Autodesk Inventor part; units mm, degrees
(part 6 of 7)
sketch "スケッチ11" plane through (148.5, 105, 2.25) normal (0, 0, 1) x (1, 0, 0)
  circle A0 centre (0, 0) radius 2 projected
  circle A1 centre (0, 0) radius 6 projected
  circle A2 centre (0, 0) radius 18.25 projected
  arc A3 (0.4109, 20.0429) -> (0.2771, 19.6719) centre (6.369, 17.6849) ccw projected
  arc A4 (0.6052, 20.4911) -> (0.4109, 20.0429) centre (7.4658, 17.2508) ccw projected
  arc A5 (1.0044, 20.4754) -> (0.6052, 20.4911) centre (0, 0) ccw projected
  arc A6 (1.1629, 20.0133) -> (1.0044, 20.4754) centre (-6.0894, 17.7834) ccw projected
  arc A7 (1.2671, 19.633) -> (1.1629, 20.0133) centre (-4.9618, 18.1301) ccw projected
  arc A8 (1.331, 19.3292) -> (1.2671, 19.633) centre (-3.8577, 18.3965) ccw projected
  arc A9 (1.7091, 19.2995) -> (1.331, 19.3292) centre (0, 0) ccw projected
  arc A10 (1.8197, 19.5895) -> (1.7091, 19.2995) centre (6.6881, 17.5665) ccw projected
  arc A11 (1.9822, 19.9489) -> (1.8197, 19.5895) centre (7.7369, 17.1307) ccw projected
  arc A12 (2.2111, 20.3804) -> (1.9822, 19.9489) centre (8.7963, 16.6119) ccw projected
  arc A13 (2.6078, 20.3335) -> (2.2111, 20.3804) centre (0, 0) ccw projected
  arc A14 (2.7295, 19.8604) -> (2.6078, 20.3335) centre (-4.6753, 18.2064) ccw projected
  arc A15 (2.8036, 19.473) -> (2.7295, 19.8604) centre (-3.5241, 18.4635) ccw projected
  arc A16 (2.8435, 19.1652) -> (2.8036, 19.473) centre (-2.4025, 18.6425) ccw projected
  arc A17 (3.2181, 19.1059) -> (2.8435, 19.1652) centre (0, 0) ccw projected
  arc A18 (3.3511, 19.3863) -> (3.2181, 19.1059) centre (8.0457, 16.9876) ccw projected
  arc A19 (3.5413, 19.7318) -> (3.3511, 19.3863) centre (9.0571, 16.4708) ccw projected
  arc A20 (3.8033, 20.1441) -> (3.5413, 19.7318) centre (10.0726, 15.8705) ccw projected
  arc A21 (4.1951, 20.0662) -> (3.8033, 20.1441) centre (0, 0) ccw projected
  arc A22 (4.2793, 19.585) -> (4.1951, 20.0662) centre (-3.2324, 18.517) ccw projected
  arc A23 (4.3228, 19.193) -> (4.2793, 19.585) centre (-2.0646, 18.6831) ccw projected
  arc A24 (4.3384, 18.883) -> (4.3228, 19.193) centre (-0.9324, 18.7735) ccw projected
  arc A25 (4.7072, 18.7945) -> (4.3384, 18.883) centre (0, 0) ccw projected
  arc A26 (4.8618, 19.0636) -> (4.7072, 18.7945) centre (9.3537, 16.304) ccw projected
  arc A27 (5.0785, 19.3932) -> (4.8618, 19.0636) centre (10.3215, 15.7095) ccw projected
  arc A28 (5.372, 19.7836) -> (5.0785, 19.3932) centre (11.2867, 15.0313) ccw projected
  arc A29 (5.7565, 19.6752) -> (5.372, 19.7836) centre (0, 0) ccw projected
  arc A30 (5.8028, 19.1889) -> (5.7565, 19.6752) centre (-1.7696, 18.7136) ccw projected
  arc A31 (5.8154, 18.7947) -> (5.8028, 19.1889) centre (-0.5924, 18.7875) ccw projected
  arc A32 (5.8066, 18.4844) -> (5.8154, 18.7947) centre (0.5434, 18.7888) ccw projected
  arc A33 (6.1673, 18.3672) -> (5.8066, 18.4844) centre (0, 0) ccw projected
  arc A34 (6.3425, 18.6234) -> (6.1673, 18.3672) centre (10.6041, 15.5199) ccw projected
  arc A35 (6.5844, 18.9349) -> (6.3425, 18.6234) centre (11.5222, 14.8512) ccw projected
  arc A36 (6.9077, 19.3011) -> (6.5844, 18.9349) centre (12.4312, 14.0994) ccw projected
  arc A37 (7.2825, 19.1629) -> (6.9077, 19.3011) centre (0, 0) ccw projected
  arc A38 (7.2904, 18.6745) -> (7.2825, 19.1629) centre (-0.2959, 18.7947) ccw projected
  arc A39 (7.272, 18.2805) -> (7.2904, 18.6745) centre (0.8835, 18.776) ccw projected
  arc A40 (7.2389, 17.9719) -> (7.272, 18.2805) centre (2.0159, 18.6882) ccw projected
  arc A41 (7.5893, 17.8267) -> (7.2389, 17.9719) centre (0, 0) ccw projected
  arc A42 (7.7842, 18.0684) -> (7.5893, 17.8267) centre (11.7891, 14.64) ccw projected
  arc A43 (8.0497, 18.36) -> (7.7842, 18.0684) centre (12.6519, 13.9014) ccw projected
  arc A44 (8.4007, 18.6997) -> (8.0497, 18.36) centre (13.4991, 13.0806) ccw projected
  arc A45 (8.7635, 18.5324) -> (8.4007, 18.6997) centre (0, 0) ccw projected
  arc A46 (8.7331, 18.0449) -> (8.7635, 18.5324) centre (1.1796, 18.76) ccw projected
  arc A47 (8.6839, 17.6536) -> (8.7331, 18.0449) centre (2.3539, 18.6488) ccw projected
  arc A48 (8.6267, 17.3485) -> (8.6839, 17.6536) centre (3.476, 18.4724) ccw projected
  arc A49 (8.9646, 17.1763) -> (8.6267, 17.3485) centre (0, 0) ccw projected
  arc A50 (9.1778, 17.4019) -> (8.9646, 17.1763) centre (12.9014, 13.6699) ccw projected
  arc A51 (9.4654, 17.6718) -> (9.1778, 17.4019) centre (13.7036, 12.8659) ccw projected
  arc A52 (9.842, 17.9829) -> (9.4654, 17.6718) centre (14.4838, 11.9812) ccw projected
  arc A53 (10.1905, 17.7877) -> (9.842, 17.9829) centre (0, 0) ccw projected
  arc A54 (10.122, 17.3041) -> (10.1905, 17.7877) centre (2.6478, 18.6096) ccw projected
  arc A55 (10.0422, 16.9178) -> (10.122, 17.3041) centre (3.8099, 18.4067) ccw projected
  arc A56 (9.9612, 16.6182) -> (10.0422, 16.9178) centre (4.9146, 18.1428) ccw projected
  arc A57 (10.2846, 16.42) -> (9.9612, 16.6182) centre (0, 0) ccw projected
  arc A58 (10.5148, 16.6282) -> (10.2846, 16.42) centre (13.9341, 12.6156) ccw projected
  arc A59 (10.8227, 16.8747) -> (10.5148, 16.6282) centre (14.6708, 11.7511) ccw projected
  arc A60 (11.2226, 17.1553) -> (10.8227, 16.8747) centre (15.3792, 10.8078) ccw projected
  arc A61 (11.5547, 16.9334) -> (11.2226, 17.1553) centre (0, 0) ccw projected
  arc A62 (11.4485, 16.4566) -> (11.5547, 16.9334) centre (4.0998, 18.3445) ccw projected
  arc A63 (11.3386, 16.0778) -> (11.4485, 16.4566) centre (5.2423, 18.051) ccw projected
  arc A64 (11.2344, 15.7854) -> (11.3386, 16.0778) centre (6.3229, 17.7012) ccw projected
  arc A65 (11.5412, 15.5625) -> (11.2344, 15.7854) centre (0, 0) ccw projected
  arc A66 (11.7871, 15.752) -> (11.5412, 15.5625) centre (14.881, 11.4834) ccw projected
  arc A67 (12.1134, 15.9735) -> (11.7871, 15.752) centre (15.5476, 10.5638) ccw projected
  arc A68 (12.534, 16.2219) -> (12.1134, 15.9735) centre (16.1798, 9.5679) ccw projected
  arc A69 (12.8477, 15.9746) -> (12.534, 16.2219) centre (0, 0) ccw projected
  arc A70 (12.7043, 15.5076) -> (12.8477, 15.9746) centre (5.5264, 17.9663) ccw projected
  arc A71 (12.5651, 15.1386) -> (12.7043, 15.5076) centre (6.6424, 17.5841) ccw projected
  arc A72 (12.4383, 14.8553) -> (12.5651, 15.1386) centre (7.6922, 17.1506) ccw projected
  arc A73 (12.7266, 14.609) -> (12.4383, 14.8553) centre (0, 0) ccw projected
  arc A74 (12.9866, 14.7786) -> (12.7266, 14.609) centre (15.7361, 10.2805) ccw projected
  arc A75 (13.3293, 14.9739) -> (12.9866, 14.7786) centre (16.3285, 9.3114) ccw projected
  arc A76 (13.7681, 15.1885) -> (13.3293, 14.9739) centre (16.8806, 8.2689) ccw projected
  arc A77 (14.0614, 14.9173) -> (13.7681, 15.1885) centre (0, 0) ccw projected
  arc A78 (13.8819, 14.463) -> (14.0614, 14.9173) centre (6.919, 17.4773) ccw projected
  arc A79 (13.7141, 14.1061) -> (13.8819, 14.463) centre (8.0015, 17.0087) ccw projected
  arc A80 (13.5655, 13.8336) -> (13.7141, 14.1061) centre (9.0141, 16.4942) ccw projected
  arc A81 (13.8336, 13.5655) -> (13.5655, 13.8336) centre (0, 0) ccw projected
  arc A82 (14.1061, 13.7141) -> (13.8336, 13.5655) centre (16.4942, 9.0141) ccw projected
  arc A83 (14.463, 13.8819) -> (14.1061, 13.7141) centre (17.0087, 8.0015) ccw projected
  arc A84 (14.9173, 14.0614) -> (14.463, 13.8819) centre (17.4773, 6.919) ccw projected
  arc A85 (15.1885, 13.7681) -> (14.9173, 14.0614) centre (0, 0) ccw projected
  arc A86 (14.9739, 13.3293) -> (15.1885, 13.7681) centre (8.2689, 16.8806) ccw projected
  arc A87 (14.7786, 12.9866) -> (14.9739, 13.3293) centre (9.3114, 16.3285) ccw projected
  arc A88 (14.609, 12.7266) -> (14.7786, 12.9866) centre (10.2805, 15.7361) ccw projected
  arc A89 (14.8553, 12.4383) -> (14.609, 12.7266) centre (0, 0) ccw projected
  arc A90 (15.1386, 12.5651) -> (14.8553, 12.4383) centre (17.1506, 7.6922) ccw projected
  arc A91 (15.5076, 12.7043) -> (15.1386, 12.5651) centre (17.5841, 6.6424) ccw projected
  arc A92 (15.9746, 12.8477) -> (15.5076, 12.7043) centre (17.9663, 5.5264) ccw projected
  arc A93 (16.2219, 12.534) -> (15.9746, 12.8477) centre (0, 0) ccw projected
  arc A94 (15.9735, 12.1134) -> (16.2219, 12.534) centre (9.5679, 16.1798) ccw projected
  arc A95 (15.752, 11.7871) -> (15.9735, 12.1134) centre (10.5638, 15.5476) ccw projected
  arc A96 (15.5625, 11.5412) -> (15.752, 11.7871) centre (11.4834, 14.881) ccw projected
  arc A97 (15.7854, 11.2344) -> (15.5625, 11.5412) centre (0, 0) ccw projected
  arc A98 (16.0778, 11.3386) -> (15.7854, 11.2344) centre (17.7012, 6.3229) ccw projected
  arc A99 (16.4566, 11.4485) -> (16.0778, 11.3386) centre (18.051, 5.2423) ccw projected
  arc A100 (16.9334, 11.5547) -> (16.4566, 11.4485) centre (18.3445, 4.0998) ccw projected
  arc A101 (17.1553, 11.2226) -> (16.9334, 11.5547) centre (0, 0) ccw projected
  arc A102 (16.8747, 10.8227) -> (17.1553, 11.2226) centre (10.8078, 15.3792) ccw projected
  arc A103 (16.6282, 10.5148) -> (16.8747, 10.8227) centre (11.7511, 14.6708) ccw projected
  arc A104 (16.42, 10.2846) -> (16.6282, 10.5148) centre (12.6156, 13.9341) ccw projected
  arc A105 (16.6182, 9.9612) -> (16.42, 10.2846) centre (0, 0) ccw projected
  arc A106 (16.9178, 10.0422) -> (16.6182, 9.9612) centre (18.1428, 4.9146) ccw projected
  arc A107 (17.3041, 10.122) -> (16.9178, 10.0422) centre (18.4067, 3.8099) ccw projected
  arc A108 (17.7877, 10.1905) -> (17.3041, 10.122) centre (18.6096, 2.6478) ccw projected
  arc A109 (17.9829, 9.842) -> (17.7877, 10.1905) centre (0, 0) ccw projected
  arc A110 (17.6718, 9.4654) -> (17.9829, 9.842) centre (11.9812, 14.4838) ccw projected
  arc A111 (17.4019, 9.1778) -> (17.6718, 9.4654) centre (12.8659, 13.7036) ccw projected
  arc A112 (17.1763, 8.9646) -> (17.4019, 9.1778) centre (13.6699, 12.9014) ccw projected
  arc A113 (17.3485, 8.6267) -> (17.1763, 8.9646) centre (0, 0) ccw projected
  arc A114 (17.6536, 8.6839) -> (17.3485, 8.6267) centre (18.4724, 3.476) ccw projected
  arc A115 (18.0449, 8.7331) -> (17.6536, 8.6839) centre (18.6488, 2.3539) ccw projected
  arc A116 (18.5324, 8.7635) -> (18.0449, 8.7331) centre (18.76, 1.1796) ccw projected
  arc A117 (18.6997, 8.4007) -> (18.5324, 8.7635) centre (0, 0) ccw projected
  arc A118 (18.36, 8.0497) -> (18.6997, 8.4007) centre (13.0806, 13.4991) ccw projected
  arc A119 (18.0684, 7.7842) -> (18.36, 8.0497) centre (13.9014, 12.6519) ccw projected
  arc A120 (17.8267, 7.5893) -> (18.0684, 7.7842) centre (14.64, 11.7891) ccw projected
  arc A121 (17.9719, 7.2389) -> (17.8267, 7.5893) centre (0, 0) ccw projected
  arc A122 (18.2805, 7.272) -> (17.9719, 7.2389) centre (18.6882, 2.0159) ccw projected
  arc A123 (18.6745, 7.2904) -> (18.2805, 7.272) centre (18.776, 0.8835) ccw projected
  arc A124 (19.1629, 7.2825) -> (18.6745, 7.2904) centre (18.7947, -0.2959) ccw projected
  arc A125 (19.3011, 6.9077) -> (19.1629, 7.2825) centre (0, 0) ccw projected
  arc A126 (18.9349, 6.5844) -> (19.3011, 6.9077) centre (14.0994, 12.4312) ccw projected
  arc A127 (18.6234, 6.3425) -> (18.9349, 6.5844) centre (14.8512, 11.5222) ccw projected
  arc A128 (18.3672, 6.1673) -> (18.6234, 6.3425) centre (15.5199, 10.6041) ccw projected
  arc A129 (18.4844, 5.8066) -> (18.3672, 6.1673) centre (0, 0) ccw projected
  arc A130 (18.7947, 5.8154) -> (18.4844, 5.8066) centre (18.7888, 0.5434) ccw projected
  arc A131 (19.1889, 5.8028) -> (18.7947, 5.8154) centre (18.7875, -0.5924) ccw projected
  arc A132 (19.6752, 5.7565) -> (19.1889, 5.8028) centre (18.7136, -1.7696) ccw projected
  arc A133 (19.7836, 5.372) -> (19.6752, 5.7565) centre (0, 0) ccw projected
  arc A134 (19.3932, 5.0785) -> (19.7836, 5.372) centre (15.0313, 11.2867) ccw projected
  arc A135 (19.0636, 4.8618) -> (19.3932, 5.0785) centre (15.7095, 10.3215) ccw projected
  arc A136 (18.7945, 4.7072) -> (19.0636, 4.8618) centre (16.304, 9.3537) ccw projected
  arc A137 (18.883, 4.3384) -> (18.7945, 4.7072) centre (0, 0) ccw projected
  arc A138 (19.193, 4.3228) -> (18.883, 4.3384) centre (18.7735, -0.9324) ccw projected
  arc A139 (19.585, 4.2793) -> (19.193, 4.3228) centre (18.6831, -2.0646) ccw projected
  arc A140 (20.0662, 4.1951) -> (19.585, 4.2793) centre (18.517, -3.2324) ccw projected
  arc A141 (20.1441, 3.8033) -> (20.0662, 4.1951) centre (0, 0) ccw projected
  arc A142 (19.7318, 3.5413) -> (20.1441, 3.8033) centre (15.8705, 10.0726) ccw projected
  arc A143 (19.3863, 3.3511) -> (19.7318, 3.5413) centre (16.4708, 9.0571) ccw projected
  arc A144 (19.1059, 3.2181) -> (19.3863, 3.3511) centre (16.9876, 8.0457) ccw projected
  arc A145 (19.1652, 2.8435) -> (19.1059, 3.2181) centre (0, 0) ccw projected
  arc A146 (19.473, 2.8036) -> (19.1652, 2.8435) centre (18.6425, -2.4025) ccw projected
  arc A147 (19.8604, 2.7295) -> (19.473, 2.8036) centre (18.4635, -3.5241) ccw projected
  arc A148 (20.3335, 2.6078) -> (19.8604, 2.7295) centre (18.2064, -4.6753) ccw projected
  arc A149 (20.3804, 2.2111) -> (20.3335, 2.6078) centre (0, 0) ccw projected
  arc A150 (19.9489, 1.9822) -> (20.3804, 2.2111) centre (16.6119, 8.7963) ccw projected
  arc A151 (19.5895, 1.8197) -> (19.9489, 1.9822) centre (17.1307, 7.7369) ccw projected
  arc A152 (19.2995, 1.7091) -> (19.5895, 1.8197) centre (17.5665, 6.6881) ccw projected
  arc A153 (19.3292, 1.331) -> (19.2995, 1.7091) centre (0, 0) ccw projected
  arc A154 (19.633, 1.2671) -> (19.3292, 1.331) centre (18.3965, -3.8577) ccw projected
  arc A155 (20.0133, 1.1629) -> (19.633, 1.2671) centre (18.1301, -4.9618) ccw projected
  arc A156 (20.4754, 1.0044) -> (20.0133, 1.1629) centre (17.7834, -6.0894) ccw projected
  arc A157 (20.4911, 0.6052) -> (20.4754, 1.0044) centre (0, 0) ccw projected
  arc A158 (20.0429, 0.4109) -> (20.4911, 0.6052) centre (17.2508, 7.4658) ccw projected
  arc A159 (19.6719, 0.2771) -> (20.0429, 0.4109) centre (17.6849, 6.369) ccw projected
  arc A160 (19.3741, 0.1896) -> (19.6719, 0.2771) centre (18.0371, 5.2892) ccw projected
  arc A161 (19.3741, -0.1896) -> (19.3741, 0.1896) centre (0, 0) ccw projected
  arc A162 (19.6719, -0.2771) -> (19.3741, -0.1896) centre (18.0371, -5.2892) ccw projected
  arc A163 (20.0429, -0.4109) -> (19.6719, -0.2771) centre (17.6849, -6.369) ccw projected
  arc A164 (20.4911, -0.6052) -> (20.0429, -0.4109) centre (17.2508, -7.4658) ccw projected
  arc A165 (20.4754, -1.0044) -> (20.4911, -0.6052) centre (0, 0) ccw projected
  arc A166 (20.0133, -1.1629) -> (20.4754, -1.0044) centre (17.7834, 6.0894) ccw projected
  arc A167 (19.633, -1.2671) -> (20.0133, -1.1629) centre (18.1301, 4.9618) ccw projected
  arc A168 (19.3292, -1.331) -> (19.633, -1.2671) centre (18.3965, 3.8577) ccw projected
  arc A169 (19.2995, -1.7091) -> (19.3292, -1.331) centre (0, 0) ccw projected
  arc A170 (19.5895, -1.8197) -> (19.2995, -1.7091) centre (17.5665, -6.6881) ccw projected
  arc A171 (19.9489, -1.9822) -> (19.5895, -1.8197) centre (17.1307, -7.7369) ccw projected
  arc A172 (20.3804, -2.2111) -> (19.9489, -1.9822) centre (16.6119, -8.7963) ccw projected
  arc A173 (20.3335, -2.6078) -> (20.3804, -2.2111) centre (0, 0) ccw projected
  arc A174 (19.8604, -2.7295) -> (20.3335, -2.6078) centre (18.2064, 4.6753) ccw projected
  arc A175 (19.473, -2.8036) -> (19.8604, -2.7295) centre (18.4635, 3.5241) ccw projected
  arc A176 (19.1652, -2.8435) -> (19.473, -2.8036) centre (18.6425, 2.4025) ccw projected
  arc A177 (19.1059, -3.2181) -> (19.1652, -2.8435) centre (0, 0) ccw projected
  arc A178 (19.3863, -3.3511) -> (19.1059, -3.2181) centre (16.9876, -8.0457) ccw projected
  arc A179 (19.7318, -3.5413) -> (19.3863, -3.3511) centre (16.4708, -9.0571) ccw projected
  arc A180 (20.1441, -3.8033) -> (19.7318, -3.5413) centre (15.8705, -10.0726) ccw projected
  arc A181 (20.0662, -4.1951) -> (20.1441, -3.8033) centre (0, 0) ccw projected
  arc A182 (19.585, -4.2793) -> (20.0662, -4.1951) centre (18.517, 3.2324) ccw projected
  arc A183 (19.193, -4.3228) -> (19.585, -4.2793) centre (18.6831, 2.0646) ccw projected
  arc A184 (18.883, -4.3384) -> (19.193, -4.3228) centre (18.7735, 0.9324) ccw projected
  arc A185 (18.7945, -4.7072) -> (18.883, -4.3384) centre (0, 0) ccw projected
  arc A186 (19.0636, -4.8618) -> (18.7945, -4.7072) centre (16.304, -9.3537) ccw projected
  arc A187 (19.3932, -5.0785) -> (19.0636, -4.8618) centre (15.7095, -10.3215) ccw projected
  arc A188 (19.7836, -5.372) -> (19.3932, -5.0785) centre (15.0313, -11.2867) ccw projected
  arc A189 (19.6752, -5.7565) -> (19.7836, -5.372) centre (0, 0) ccw projected
  arc A190 (19.1889, -5.8028) -> (19.6752, -5.7565) centre (18.7136, 1.7696) ccw projected
  arc A191 (18.7947, -5.8154) -> (19.1889, -5.8028) centre (18.7875, 0.5924) ccw projected
  arc A192 (18.4844, -5.8066) -> (18.7947, -5.8154) centre (18.7888, -0.5434) ccw projected
  arc A193 (18.3672, -6.1673) -> (18.4844, -5.8066) centre (0, 0) ccw projected
  arc A194 (18.6234, -6.3425) -> (18.3672, -6.1673) centre (15.5199, -10.6041) ccw projected
  arc A195 (18.9349, -6.5844) -> (18.6234, -6.3425) centre (14.8512, -11.5222) ccw projected
  arc A196 (19.3011, -6.9077) -> (18.9349, -6.5844) centre (14.0994, -12.4312) ccw projected
  arc A197 (19.1629, -7.2825) -> (19.3011, -6.9077) centre (0, 0) ccw projected
  arc A198 (18.6745, -7.2904) -> (19.1629, -7.2825) centre (18.7947, 0.2959) ccw projected
  arc A199 (18.2805, -7.272) -> (18.6745, -7.2904) centre (18.776, -0.8835) ccw projected
  arc A200 (17.9719, -7.2389) -> (18.2805, -7.272) centre (18.6882, -2.0159) ccw projected
  arc A201 (17.8267, -7.5893) -> (17.9719, -7.2389) centre (0, 0) ccw projected
  arc A202 (18.0684, -7.7842) -> (17.8267, -7.5893) centre (14.64, -11.7891) ccw projected
  arc A203 (18.36, -8.0497) -> (18.0684, -7.7842) centre (13.9014, -12.6519) ccw projected
  arc A204 (18.6997, -8.4007) -> (18.36, -8.0497) centre (13.0806, -13.4991) ccw projected
  arc A205 (18.5324, -8.7635) -> (18.6997, -8.4007) centre (0, 0) ccw projected
  arc A206 (18.0449, -8.7331) -> (18.5324, -8.7635) centre (18.76, -1.1796) ccw projected
  arc A207 (17.6536, -8.6839) -> (18.0449, -8.7331) centre (18.6488, -2.3539) ccw projected
  arc A208 (17.3485, -8.6267) -> (17.6536, -8.6839) centre (18.4724, -3.476) ccw projected
  arc A209 (17.1763, -8.9646) -> (17.3485, -8.6267) centre (0, 0) ccw projected
  arc A210 (17.4019, -9.1778) -> (17.1763, -8.9646) centre (13.6699, -12.9014) ccw projected
  arc A211 (17.6718, -9.4654) -> (17.4019, -9.1778) centre (12.8659, -13.7036) ccw projected
  arc A212 (17.9829, -9.842) -> (17.6718, -9.4654) centre (11.9812, -14.4838) ccw projected
  arc A213 (17.7877, -10.1905) -> (17.9829, -9.842) centre (0, 0) ccw projected
  arc A214 (17.3041, -10.122) -> (17.7877, -10.1905) centre (18.6096, -2.6478) ccw projected
  arc A215 (16.9178, -10.0422) -> (17.3041, -10.122) centre (18.4067, -3.8099) ccw projected
  arc A216 (16.6182, -9.9612) -> (16.9178, -10.0422) centre (18.1428, -4.9146) ccw projected
  arc A217 (16.42, -10.2846) -> (16.6182, -9.9612) centre (0, 0) ccw projected
  arc A218 (16.6282, -10.5148) -> (16.42, -10.2846) centre (12.6156, -13.9341) ccw projected
  arc A219 (16.8747, -10.8227) -> (16.6282, -10.5148) centre (11.7511, -14.6708) ccw projected
  arc A220 (17.1553, -11.2226) -> (16.8747, -10.8227) centre (10.8078, -15.3792) ccw projected
  arc A221 (16.9334, -11.5547) -> (17.1553, -11.2226) centre (0, 0) ccw projected
  arc A222 (16.4566, -11.4485) -> (16.9334, -11.5547) centre (18.3445, -4.0998) ccw projected
  arc A223 (16.0778, -11.3386) -> (16.4566, -11.4485) centre (18.051, -5.2423) ccw projected
  arc A224 (15.7854, -11.2344) -> (16.0778, -11.3386) centre (17.7012, -6.3229) ccw projected
  arc A225 (15.5625, -11.5412) -> (15.7854, -11.2344) centre (0, 0) ccw projected
  arc A226 (15.752, -11.7871) -> (15.5625, -11.5412) centre (11.4834, -14.881) ccw projected
  arc A227 (15.9735, -12.1134) -> (15.752, -11.7871) centre (10.5638, -15.5476) ccw projected
  arc A228 (16.2219, -12.534) -> (15.9735, -12.1134) centre (9.5679, -16.1798) ccw projected
  arc A229 (15.9746, -12.8477) -> (16.2219, -12.534) centre (0, 0) ccw projected
  arc A230 (15.5076, -12.7043) -> (15.9746, -12.8477) centre (17.9663, -5.5264) ccw projected
  arc A231 (15.1386, -12.5651) -> (15.5076, -12.7043) centre (17.5841, -6.6424) ccw projected
  arc A232 (14.8553, -12.4383) -> (15.1386, -12.5651) centre (17.1506, -7.6922) ccw projected
  arc A233 (14.609, -12.7266) -> (14.8553, -12.4383) centre (0, 0) ccw projected
  arc A234 (14.7786, -12.9866) -> (14.609, -12.7266) centre (10.2805, -15.7361) ccw projected
  arc A235 (14.9739, -13.3293) -> (14.7786, -12.9866) centre (9.3114, -16.3285) ccw projected
  arc A236 (15.1885, -13.7681) -> (14.9739, -13.3293) centre (8.2689, -16.8806) ccw projected
  arc A237 (14.9173, -14.0614) -> (15.1885, -13.7681) centre (0, 0) ccw projected
  arc A238 (14.463, -13.8819) -> (14.9173, -14.0614) centre (17.4773, -6.919) ccw projected
  arc A239 (14.1061, -13.7141) -> (14.463, -13.8819) centre (17.0087, -8.0015) ccw projected
  arc A240 (13.8336, -13.5655) -> (14.1061, -13.7141) centre (16.4942, -9.0141) ccw projected
  arc A241 (13.5655, -13.8336) -> (13.8336, -13.5655) centre (0, 0) ccw projected
  arc A242 (13.7141, -14.1061) -> (13.5655, -13.8336) centre (9.0141, -16.4942) ccw projected
  arc A243 (13.8819, -14.463) -> (13.7141, -14.1061) centre (8.0015, -17.0087) ccw projected
  arc A244 (14.0614, -14.9173) -> (13.8819, -14.463) centre (6.919, -17.4773) ccw projected
  arc A245 (13.7681, -15.1885) -> (14.0614, -14.9173) centre (0, 0) ccw projected
  arc A246 (13.3293, -14.9739) -> (13.7681, -15.1885) centre (16.8806, -8.2689) ccw projected
  arc A247 (12.9866, -14.7786) -> (13.3293, -14.9739) centre (16.3285, -9.3114) ccw projected
  arc A248 (12.7266, -14.609) -> (12.9866, -14.7786) centre (15.7361, -10.2805) ccw projected
  arc A249 (12.4383, -14.8553) -> (12.7266, -14.609) centre (0, 0) ccw projected
  arc A250 (12.5651, -15.1386) -> (12.4383, -14.8553) centre (7.6922, -17.1506) ccw projected
  arc A251 (12.7043, -15.5076) -> (12.5651, -15.1386) centre (6.6424, -17.5841) ccw projected
  arc A252 (12.8477, -15.9746) -> (12.7043, -15.5076) centre (5.5264, -17.9663) ccw projected
  arc A253 (12.534, -16.2219) -> (12.8477, -15.9746) centre (0, 0) ccw projected
  arc A254 (12.1134, -15.9735) -> (12.534, -16.2219) centre (16.1798, -9.5679) ccw projected
  arc A255 (11.7871, -15.752) -> (12.1134, -15.9735) centre (15.5476, -10.5638) ccw projected
  arc A256 (11.5412, -15.5625) -> (11.7871, -15.752) centre (14.881, -11.4834) ccw projected
  arc A257 (11.2344, -15.7854) -> (11.5412, -15.5625) centre (0, 0) ccw projected
  arc A258 (11.3386, -16.0778) -> (11.2344, -15.7854) centre (6.3229, -17.7012) ccw projected
  arc A259 (11.4485, -16.4566) -> (11.3386, -16.0778) centre (5.2423, -18.051) ccw projected
  arc A260 (11.5547, -16.9334) -> (11.4485, -16.4566) centre (4.0998, -18.3445) ccw projected
  arc A261 (11.2226, -17.1553) -> (11.5547, -16.9334) centre (0, 0) ccw projected
  arc A262 (10.8227, -16.8747) -> (11.2226, -17.1553) centre (15.3792, -10.8078) ccw projected
  arc A263 (10.5148, -16.6282) -> (10.8227, -16.8747) centre (14.6708, -11.7511) ccw projected
  arc A264 (10.2846, -16.42) -> (10.5148, -16.6282) centre (13.9341, -12.6156) ccw projected
  arc A265 (9.9612, -16.6182) -> (10.2846, -16.42) centre (0, 0) ccw projected
  arc A266 (10.0422, -16.9178) -> (9.9612, -16.6182) centre (4.9146, -18.1428) ccw projected
  arc A267 (10.122, -17.3041) -> (10.0422, -16.9178) centre (3.8099, -18.4067) ccw projected
  arc A268 (10.1905, -17.7877) -> (10.122, -17.3041) centre (2.6478, -18.6096) ccw projected
  arc A269 (9.842, -17.9829) -> (10.1905, -17.7877) centre (0, 0) ccw projected
  arc A270 (9.4654, -17.6718) -> (9.842, -17.9829) centre (14.4838, -11.9812) ccw projected
  arc A271 (9.1778, -17.4019) -> (9.4654, -17.6718) centre (13.7036, -12.8659) ccw projected
  arc A272 (8.9646, -17.1763) -> (9.1778, -17.4019) centre (12.9014, -13.6699) ccw projected
  arc A273 (8.6267, -17.3485) -> (8.9646, -17.1763) centre (0, 0) ccw projected
  arc A274 (8.6839, -17.6536) -> (8.6267, -17.3485) centre (3.476, -18.4724) ccw projected
  arc A275 (8.7331, -18.0449) -> (8.6839, -17.6536) centre (2.3539, -18.6488) ccw projected
  arc A276 (8.7635, -18.5324) -> (8.7331, -18.0449) centre (1.1796, -18.76) ccw projected
  arc A277 (8.4007, -18.6997) -> (8.7635, -18.5324) centre (0, 0) ccw projected
  arc A278 (8.0497, -18.36) -> (8.4007, -18.6997) centre (13.4991, -13.0806) ccw projected
  arc A279 (7.7842, -18.0684) -> (8.0497, -18.36) centre (12.6519, -13.9014) ccw projected
  arc A280 (7.5893, -17.8267) -> (7.7842, -18.0684) centre (11.7891, -14.64) ccw projected
  arc A281 (7.2389, -17.9719) -> (7.5893, -17.8267) centre (0, 0) ccw projected
  arc A282 (7.272, -18.2805) -> (7.2389, -17.9719) centre (2.0159, -18.6882) ccw projected
  arc A283 (7.2904, -18.6745) -> (7.272, -18.2805) centre (0.8835, -18.776) ccw projected
  arc A284 (7.2825, -19.1629) -> (7.2904, -18.6745) centre (-0.2959, -18.7947) ccw projected
  arc A285 (6.9077, -19.3011) -> (7.2825, -19.1629) centre (0, 0) ccw projected
  arc A286 (6.5844, -18.9349) -> (6.9077, -19.3011) centre (12.4312, -14.0994) ccw projected
  arc A287 (6.3425, -18.6234) -> (6.5844, -18.9349) centre (11.5222, -14.8512) ccw projected
  arc A288 (6.1673, -18.3672) -> (6.3425, -18.6234) centre (10.6041, -15.5199) ccw projected
  arc A289 (5.8066, -18.4844) -> (6.1673, -18.3672) centre (0, 0) ccw projected
  arc A290 (5.8154, -18.7947) -> (5.8066, -18.4844) centre (0.5434, -18.7888) ccw projected
  arc A291 (5.8028, -19.1889) -> (5.8154, -18.7947) centre (-0.5924, -18.7875) ccw projected
  arc A292 (5.7565, -19.6752) -> (5.8028, -19.1889) centre (-1.7696, -18.7136) ccw projected
  arc A293 (5.372, -19.7836) -> (5.7565, -19.6752) centre (0, 0) ccw projected
  arc A294 (5.0785, -19.3932) -> (5.372, -19.7836) centre (11.2867, -15.0313) ccw projected
  arc A295 (4.8618, -19.0636) -> (5.0785, -19.3932) centre (10.3215, -15.7095) ccw projected
  arc A296 (4.7072, -18.7945) -> (4.8618, -19.0636) centre (9.3537, -16.304) ccw projected
  arc A297 (4.3384, -18.883) -> (4.7072, -18.7945) centre (0, 0) ccw projected
  arc A298 (4.3228, -19.193) -> (4.3384, -18.883) centre (-0.9324, -18.7735) ccw projected
  arc A299 (4.2793, -19.585) -> (4.3228, -19.193) centre (-2.0646, -18.6831) ccw projected
  arc A300 (4.1951, -20.0662) -> (4.2793, -19.585) centre (-3.2324, -18.517) ccw projected
  arc A301 (3.8033, -20.1441) -> (4.1951, -20.0662) centre (0, 0) ccw projected
  arc A302 (3.5413, -19.7318) -> (3.8033, -20.1441) centre (10.0726, -15.8705) ccw projected
  arc A303 (3.3511, -19.3863) -> (3.5413, -19.7318) centre (9.0571, -16.4708) ccw projected
  arc A304 (3.2181, -19.1059) -> (3.3511, -19.3863) centre (8.0457, -16.9876) ccw projected
  arc A305 (2.8435, -19.1652) -> (3.2181, -19.1059) centre (0, 0) ccw projected
  arc A306 (2.8036, -19.473) -> (2.8435, -19.1652) centre (-2.4025, -18.6425) ccw projected
  arc A307 (2.7295, -19.8604) -> (2.8036, -19.473) centre (-3.5241, -18.4635) ccw projected
  arc A308 (2.6078, -20.3335) -> (2.7295, -19.8604) centre (-4.6753, -18.2064) ccw projected
  arc A309 (2.2111, -20.3804) -> (2.6078, -20.3335) centre (0, 0) ccw projected
  arc A310 (1.9822, -19.9489) -> (2.2111, -20.3804) centre (8.7963, -16.6119) ccw projected
  arc A311 (1.8197, -19.5895) -> (1.9822, -19.9489) centre (7.7369, -17.1307) ccw projected
  arc A312 (1.7091, -19.2995) -> (1.8197, -19.5895) centre (6.6881, -17.5665) ccw projected
  arc A313 (1.331, -19.3292) -> (1.7091, -19.2995) centre (0, 0) ccw projected
  arc A314 (1.2671, -19.633) -> (1.331, -19.3292) centre (-3.8577, -18.3965) ccw projected
  arc A315 (1.1629, -20.0133) -> (1.2671, -19.633) centre (-4.9618, -18.1301) ccw projected
  arc A316 (1.0044, -20.4754) -> (1.1629, -20.0133) centre (-6.0894, -17.7834) ccw projected
  arc A317 (0.6052, -20.4911) -> (1.0044, -20.4754) centre (0, 0) ccw projected
  arc A318 (0.4109, -20.0429) -> (0.6052, -20.4911) centre (7.4658, -17.2508) ccw projected
  arc A319 (0.2771, -19.6719) -> (0.4109, -20.0429) centre (6.369, -17.6849) ccw projected
  arc A320 (0.1896, -19.3741) -> (0.2771, -19.6719) centre (5.2892, -18.0371) ccw projected
  arc A321 (-0.1896, -19.3741) -> (0.1896, -19.3741) centre (0, 0) ccw projected
  arc A322 (-0.2771, -19.6719) -> (-0.1896, -19.3741) centre (-5.2892, -18.0371) ccw projected
  arc A323 (-0.4109, -20.0429) -> (-0.2771, -19.6719) centre (-6.369, -17.6849) ccw projected
  arc A324 (-0.6052, -20.4911) -> (-0.4109, -20.0429) centre (-7.4658, -17.2508) ccw projected
  arc A325 (-1.0044, -20.4754) -> (-0.6052, -20.4911) centre (0, 0) ccw projected
  arc A326 (-1.1629, -20.0133) -> (-1.0044, -20.4754) centre (6.0894, -17.7834) ccw projected
  arc A327 (-1.2671, -19.633) -> (-1.1629, -20.0133) centre (4.9618, -18.1301) ccw projected
  arc A328 (-1.331, -19.3292) -> (-1.2671, -19.633) centre (3.8577, -18.3965) ccw projected
  arc A329 (-1.7091, -19.2995) -> (-1.331, -19.3292) centre (0, 0) ccw projected
  arc A330 (-1.8197, -19.5895) -> (-1.7091, -19.2995) centre (-6.6881, -17.5665) ccw projected
  arc A331 (-1.9822, -19.9489) -> (-1.8197, -19.5895) centre (-7.7369, -17.1307) ccw projected
  arc A332 (-2.2111, -20.3804) -> (-1.9822, -19.9489) centre (-8.7963, -16.6119) ccw projected
  arc A333 (-2.6078, -20.3335) -> (-2.2111, -20.3804) centre (0, 0) ccw projected
  arc A334 (-2.7295, -19.8604) -> (-2.6078, -20.3335) centre (4.6753, -18.2064) ccw projected
  arc A335 (-2.8036, -19.473) -> (-2.7295, -19.8604) centre (3.5241, -18.4635) ccw projected
  arc A336 (-2.8435, -19.1652) -> (-2.8036, -19.473) centre (2.4025, -18.6425) ccw projected
  arc A337 (-3.2181, -19.1059) -> (-2.8435, -19.1652) centre (0, 0) ccw projected
  arc A338 (-3.3511, -19.3863) -> (-3.2181, -19.1059) centre (-8.0457, -16.9876) ccw projected
  arc A339 (-3.5413, -19.7318) -> (-3.3511, -19.3863) centre (-9.0571, -16.4708) ccw projected
  arc A340 (-3.8033, -20.1441) -> (-3.5413, -19.7318) centre (-10.0726, -15.8705) ccw projected
  arc A341 (-4.1951, -20.0662) -> (-3.8033, -20.1441) centre (0, 0) ccw projected
  arc A342 (-4.2793, -19.585) -> (-4.1951, -20.0662) centre (3.2324, -18.517) ccw projected
  arc A343 (-4.3228, -19.193) -> (-4.2793, -19.585) centre (2.0646, -18.6831) ccw projected
  arc A344 (-4.3384, -18.883) -> (-4.3228, -19.193) centre (0.9324, -18.7735) ccw projected
  arc A345 (-4.7072, -18.7945) -> (-4.3384, -18.883) centre (0, 0) ccw projected
  arc A346 (-4.8618, -19.0636) -> (-4.7072, -18.7945) centre (-9.3537, -16.304) ccw projected
  arc A347 (-5.0785, -19.3932) -> (-4.8618, -19.0636) centre (-10.3215, -15.7095) ccw projected
  arc A348 (-5.372, -19.7836) -> (-5.0785, -19.3932) centre (-11.2867, -15.0313) ccw projected
  arc A349 (-5.7565, -19.6752) -> (-5.372, -19.7836) centre (0, 0) ccw projected
  arc A350 (-5.8028, -19.1889) -> (-5.7565, -19.6752) centre (1.7696, -18.7136) ccw projected
  arc A351 (-5.8154, -18.7947) -> (-5.8028, -19.1889) centre (0.5924, -18.7875) ccw projected
  arc A352 (-5.8066, -18.4844) -> (-5.8154, -18.7947) centre (-0.5434, -18.7888) ccw projected
  arc A353 (-6.1673, -18.3672) -> (-5.8066, -18.4844) centre (0, 0) ccw projected
  arc A354 (-6.3425, -18.6234) -> (-6.1673, -18.3672) centre (-10.6041, -15.5199) ccw projected
  arc A355 (-6.5844, -18.9349) -> (-6.3425, -18.6234) centre (-11.5222, -14.8512) ccw projected
  arc A356 (-6.9077, -19.3011) -> (-6.5844, -18.9349) centre (-12.4312, -14.0994) ccw projected
  arc A357 (-7.2825, -19.1629) -> (-6.9077, -19.3011) centre (0, 0) ccw projected
  arc A358 (-7.2904, -18.6745) -> (-7.2825, -19.1629) centre (0.2959, -18.7947) ccw projected
  arc A359 (-7.272, -18.2805) -> (-7.2904, -18.6745) centre (-0.8835, -18.776) ccw projected
  arc A360 (-7.2389, -17.9719) -> (-7.272, -18.2805) centre (-2.0159, -18.6882) ccw projected
  arc A361 (-7.5893, -17.8267) -> (-7.2389, -17.9719) centre (0, 0) ccw projected
  arc A362 (-7.7842, -18.0684) -> (-7.5893, -17.8267) centre (-11.7891, -14.64) ccw projected
  arc A363 (-8.0497, -18.36) -> (-7.7842, -18.0684) centre (-12.6519, -13.9014) ccw projected
  arc A364 (-8.4007, -18.6997) -> (-8.0497, -18.36) centre (-13.4991, -13.0806) ccw projected
  arc A365 (-8.7635, -18.5324) -> (-8.4007, -18.6997) centre (0, 0) ccw projected
  arc A366 (-8.7331, -18.0449) -> (-8.7635, -18.5324) centre (-1.1796, -18.76) ccw projected
  arc A367 (-8.6839, -17.6536) -> (-8.7331, -18.0449) centre (-2.3539, -18.6488) ccw projected
  arc A368 (-8.6267, -17.3485) -> (-8.6839, -17.6536) centre (-3.476, -18.4724) ccw projected
  arc A369 (-8.9646, -17.1763) -> (-8.6267, -17.3485) centre (0, 0) ccw projected
  arc A370 (-9.1778, -17.4019) -> (-8.9646, -17.1763) centre (-12.9014, -13.6699) ccw projected
  arc A371 (-9.4654, -17.6718) -> (-9.1778, -17.4019) centre (-13.7036, -12.8659) ccw projected
  arc A372 (-9.842, -17.9829) -> (-9.4654, -17.6718) centre (-14.4838, -11.9812) ccw projected
  arc A373 (-10.1905, -17.7877) -> (-9.842, -17.9829) centre (0, 0) ccw projected
  arc A374 (-10.122, -17.3041) -> (-10.1905, -17.7877) centre (-2.6478, -18.6096) ccw projected
  arc A375 (-10.0422, -16.9178) -> (-10.122, -17.3041) centre (-3.8099, -18.4067) ccw projected
  arc A376 (-9.9612, -16.6182) -> (-10.0422, -16.9178) centre (-4.9146, -18.1428) ccw projected
  arc A377 (-10.2846, -16.42) -> (-9.9612, -16.6182) centre (0, 0) ccw projected
  arc A378 (-10.5148, -16.6282) -> (-10.2846, -16.42) centre (-13.9341, -12.6156) ccw projected
  arc A379 (-10.8227, -16.8747) -> (-10.5148, -16.6282) centre (-14.6708, -11.7511) ccw projected
  arc A380 (-11.2226, -17.1553) -> (-10.8227, -16.8747) centre (-15.3792, -10.8078) ccw projected
  arc A381 (-11.5547, -16.9334) -> (-11.2226, -17.1553) centre (0, 0) ccw projected
  arc A382 (-11.4485, -16.4566) -> (-11.5547, -16.9334) centre (-4.0998, -18.3445) ccw projected
  arc A383 (-11.3386, -16.0778) -> (-11.4485, -16.4566) centre (-5.2423, -18.051) ccw projected
  arc A384 (-11.2344, -15.7854) -> (-11.3386, -16.0778) centre (-6.3229, -17.7012) ccw projected
  arc A385 (-11.5412, -15.5625) -> (-11.2344, -15.7854) centre (0, 0) ccw projected
  arc A386 (-11.7871, -15.752) -> (-11.5412, -15.5625) centre (-14.881, -11.4834) ccw projected
  arc A387 (-12.1134, -15.9735) -> (-11.7871, -15.752) centre (-15.5476, -10.5638) ccw projected
  arc A388 (-12.534, -16.2219) -> (-12.1134, -15.9735) centre (-16.1798, -9.5679) ccw projected
  arc A389 (-12.8477, -15.9746) -> (-12.534, -16.2219) centre (0, 0) ccw projected
  arc A390 (-12.7043, -15.5076) -> (-12.8477, -15.9746) centre (-5.5264, -17.9663) ccw projected
  arc A391 (-12.5651, -15.1386) -> (-12.7043, -15.5076) centre (-6.6424, -17.5841) ccw projected
  arc A392 (-12.4383, -14.8553) -> (-12.5651, -15.1386) centre (-7.6922, -17.1506) ccw projected
  arc A393 (-12.7266, -14.609) -> (-12.4383, -14.8553) centre (0, 0) ccw projected
  arc A394 (-12.9866, -14.7786) -> (-12.7266, -14.609) centre (-15.7361, -10.2805) ccw projected
  arc A395 (-13.3293, -14.9739) -> (-12.9866, -14.7786) centre (-16.3285, -9.3114) ccw projected
  arc A396 (-13.7681, -15.1885) -> (-13.3293, -14.9739) centre (-16.8806, -8.2689) ccw projected
  arc A397 (-14.0614, -14.9173) -> (-13.7681, -15.1885) centre (0, 0) ccw projected
  arc A398 (-13.8819, -14.463) -> (-14.0614, -14.9173) centre (-6.919, -17.4773) ccw projected
  arc A399 (-13.7141, -14.1061) -> (-13.8819, -14.463) centre (-8.0015, -17.0087) ccw projected
  arc A400 (-13.5655, -13.8336) -> (-13.7141, -14.1061) centre (-9.0141, -16.4942) ccw projected
  arc A401 (-13.8336, -13.5655) -> (-13.5655, -13.8336) centre (0, 0) ccw projected
  arc A402 (-14.1061, -13.7141) -> (-13.8336, -13.5655) centre (-16.4942, -9.0141) ccw projected
  arc A403 (-14.463, -13.8819) -> (-14.1061, -13.7141) centre (-17.0087, -8.0015) ccw projected
  arc A404 (-14.9173, -14.0614) -> (-14.463, -13.8819) centre (-17.4773, -6.919) ccw projected
  arc A405 (-15.1885, -13.7681) -> (-14.9173, -14.0614) centre (0, 0) ccw projected
  arc A406 (-14.9739, -13.3293) -> (-15.1885, -13.7681) centre (-8.2689, -16.8806) ccw projected
  arc A407 (-14.7786, -12.9866) -> (-14.9739, -13.3293) centre (-9.3114, -16.3285) ccw projected
  arc A408 (-14.609, -12.7266) -> (-14.7786, -12.9866) centre (-10.2805, -15.7361) ccw projected
  arc A409 (-14.8553, -12.4383) -> (-14.609, -12.7266) centre (0, 0) ccw projected
  arc A410 (-15.1386, -12.5651) -> (-14.8553, -12.4383) centre (-17.1506, -7.6922) ccw projected
  arc A411 (-15.5076, -12.7043) -> (-15.1386, -12.5651) centre (-17.5841, -6.6424) ccw projected
  arc A412 (-15.9746, -12.8477) -> (-15.5076, -12.7043) centre (-17.9663, -5.5264) ccw projected
  arc A413 (-16.2219, -12.534) -> (-15.9746, -12.8477) centre (0, 0) ccw projected
  arc A414 (-15.9735, -12.1134) -> (-16.2219, -12.534) centre (-9.5679, -16.1798) ccw projected
  arc A415 (-15.752, -11.7871) -> (-15.9735, -12.1134) centre (-10.5638, -15.5476) ccw projected
  arc A416 (-15.5625, -11.5412) -> (-15.752, -11.7871) centre (-11.4834, -14.881) ccw projected
  arc A417 (-15.7854, -11.2344) -> (-15.5625, -11.5412) centre (0, 0) ccw projected
  arc A418 (-16.0778, -11.3386) -> (-15.7854, -11.2344) centre (-17.7012, -6.3229) ccw projected
  arc A419 (-16.4566, -11.4485) -> (-16.0778, -11.3386) centre (-18.051, -5.2423) ccw projected
  arc A420 (-16.9334, -11.5547) -> (-16.4566, -11.4485) centre (-18.3445, -4.0998) ccw projected
  arc A421 (-17.1553, -11.2226) -> (-16.9334, -11.5547) centre (0, 0) ccw projected
  arc A422 (-16.8747, -10.8227) -> (-17.1553, -11.2226) centre (-10.8078, -15.3792) ccw projected
  arc A423 (-16.6282, -10.5148) -> (-16.8747, -10.8227) centre (-11.7511, -14.6708) ccw projected
  arc A424 (-16.42, -10.2846) -> (-16.6282, -10.5148) centre (-12.6156, -13.9341) ccw projected
  arc A425 (-16.6182, -9.9612) -> (-16.42, -10.2846) centre (0, 0) ccw projected
  arc A426 (-16.9178, -10.0422) -> (-16.6182, -9.9612) centre (-18.1428, -4.9146) ccw projected
  arc A427 (-17.3041, -10.122) -> (-16.9178, -10.0422) centre (-18.4067, -3.8099) ccw projected
  arc A428 (-17.7877, -10.1905) -> (-17.3041, -10.122) centre (-18.6096, -2.6478) ccw projected
  arc A429 (-17.9829, -9.842) -> (-17.7877, -10.1905) centre (0, 0) ccw projected
  arc A430 (-17.6718, -9.4654) -> (-17.9829, -9.842) centre (-11.9812, -14.4838) ccw projected
  arc A431 (-17.4019, -9.1778) -> (-17.6718, -9.4654) centre (-12.8659, -13.7036) ccw projected
  arc A432 (-17.1763, -8.9646) -> (-17.4019, -9.1778) centre (-13.6699, -12.9014) ccw projected
  arc A433 (-17.3485, -8.6267) -> (-17.1763, -8.9646) centre (0, 0) ccw projected
  arc A434 (-17.6536, -8.6839) -> (-17.3485, -8.6267) centre (-18.4724, -3.476) ccw projected
  arc A435 (-18.0449, -8.7331) -> (-17.6536, -8.6839) centre (-18.6488, -2.3539) ccw projected
  arc A436 (-18.5324, -8.7635) -> (-18.0449, -8.7331) centre (-18.76, -1.1796) ccw projected
  arc A437 (-18.6997, -8.4007) -> (-18.5324, -8.7635) centre (0, 0) ccw projected
  arc A438 (-18.36, -8.0497) -> (-18.6997, -8.4007) centre (-13.0806, -13.4991) ccw projected
  arc A439 (-18.0684, -7.7842) -> (-18.36, -8.0497) centre (-13.9014, -12.6519) ccw projected
  arc A440 (-17.8267, -7.5893) -> (-18.0684, -7.7842) centre (-14.64, -11.7891) ccw projected
  arc A441 (-17.9719, -7.2389) -> (-17.8267, -7.5893) centre (0, 0) ccw projected
  arc A442 (-18.2805, -7.272) -> (-17.9719, -7.2389) centre (-18.6882, -2.0159) ccw projected
  arc A443 (-18.6745, -7.2904) -> (-18.2805, -7.272) centre (-18.776, -0.8835) ccw projected
  arc A444 (-19.1629, -7.2825) -> (-18.6745, -7.2904) centre (-18.7947, 0.2959) ccw projected
  arc A445 (-19.3011, -6.9077) -> (-19.1629, -7.2825) centre (0, 0) ccw projected
  arc A446 (-18.9349, -6.5844) -> (-19.3011, -6.9077) centre (-14.0994, -12.4312) ccw projected
  arc A447 (-18.6234, -6.3425) -> (-18.9349, -6.5844) centre (-14.8512, -11.5222) ccw projected
  arc A448 (-18.3672, -6.1673) -> (-18.6234, -6.3425) centre (-15.5199, -10.6041) ccw projected
  arc A449 (-18.4844, -5.8066) -> (-18.3672, -6.1673) centre (0, 0) ccw projected
  arc A450 (-18.7947, -5.8154) -> (-18.4844, -5.8066) centre (-18.7888, -0.5434) ccw projected
  arc A451 (-19.1889, -5.8028) -> (-18.7947, -5.8154) centre (-18.7875, 0.5924) ccw projected
  arc A452 (-19.6752, -5.7565) -> (-19.1889, -5.8028) centre (-18.7136, 1.7696) ccw projected
  arc A453 (-19.7836, -5.372) -> (-19.6752, -5.7565) centre (0, 0) ccw projected
  arc A454 (-19.3932, -5.0785) -> (-19.7836, -5.372) centre (-15.0313, -11.2867) ccw projected
  arc A455 (-19.0636, -4.8618) -> (-19.3932, -5.0785) centre (-15.7095, -10.3215) ccw projected
  arc A456 (-18.7945, -4.7072) -> (-19.0636, -4.8618) centre (-16.304, -9.3537) ccw projected
  arc A457 (-18.883, -4.3384) -> (-18.7945, -4.7072) centre (0, 0) ccw projected
  arc A458 (-19.193, -4.3228) -> (-18.883, -4.3384) centre (-18.7735, 0.9324) ccw projected
  arc A459 (-19.585, -4.2793) -> (-19.193, -4.3228) centre (-18.6831, 2.0646) ccw projected
  arc A460 (-20.0662, -4.1951) -> (-19.585, -4.2793) centre (-18.517, 3.2324) ccw projected
  arc A461 (-20.1441, -3.8033) -> (-20.0662, -4.1951) centre (0, 0) ccw projected
  arc A462 (-19.7318, -3.5413) -> (-20.1441, -3.8033) centre (-15.8705, -10.0726) ccw projected
  arc A463 (-19.3863, -3.3511) -> (-19.7318, -3.5413) centre (-16.4708, -9.0571) ccw projected
  arc A464 (-19.1059, -3.2181) -> (-19.3863, -3.3511) centre (-16.9876, -8.0457) ccw projected
  arc A465 (-19.1652, -2.8435) -> (-19.1059, -3.2181) centre (0, 0) ccw projected
  arc A466 (-19.473, -2.8036) -> (-19.1652, -2.8435) centre (-18.6425, 2.4025) ccw projected
  arc A467 (-19.8604, -2.7295) -> (-19.473, -2.8036) centre (-18.4635, 3.5241) ccw projected
  arc A468 (-20.3335, -2.6078) -> (-19.8604, -2.7295) centre (-18.2064, 4.6753) ccw projected
  arc A469 (-20.3804, -2.2111) -> (-20.3335, -2.6078) centre (0, 0) ccw projected
  arc A470 (-19.9489, -1.9822) -> (-20.3804, -2.2111) centre (-16.6119, -8.7963) ccw projected
  arc A471 (-19.5895, -1.8197) -> (-19.9489, -1.9822) centre (-17.1307, -7.7369) ccw projected
  arc A472 (-19.2995, -1.7091) -> (-19.5895, -1.8197) centre (-17.5665, -6.6881) ccw projected
  arc A473 (-19.3292, -1.331) -> (-19.2995, -1.7091) centre (0, 0) ccw projected
  arc A474 (-19.633, -1.2671) -> (-19.3292, -1.331) centre (-18.3965, 3.8577) ccw projected
  arc A475 (-20.0133, -1.1629) -> (-19.633, -1.2671) centre (-18.1301, 4.9618) ccw projected
  arc A476 (-20.4754, -1.0044) -> (-20.0133, -1.1629) centre (-17.7834, 6.0894) ccw projected
  arc A477 (-20.4911, -0.6052) -> (-20.4754, -1.0044) centre (0, 0) ccw projected
  arc A478 (-20.0429, -0.4109) -> (-20.4911, -0.6052) centre (-17.2508, -7.4658) ccw projected
  arc A479 (-19.6719, -0.2771) -> (-20.0429, -0.4109) centre (-17.6849, -6.369) ccw projected
  arc A480 (-19.3741, -0.1896) -> (-19.6719, -0.2771) centre (-18.0371, -5.2892) ccw projected
  arc A481 (-19.3741, 0.1896) -> (-19.3741, -0.1896) centre (0, 0) ccw projected
  arc A482 (-19.6719, 0.2771) -> (-19.3741, 0.1896) centre (-18.0371, 5.2892) ccw projected
  arc A483 (-20.0429, 0.4109) -> (-19.6719, 0.2771) centre (-17.6849, 6.369) ccw projected
  arc A484 (-20.4911, 0.6052) -> (-20.0429, 0.4109) centre (-17.2508, 7.4658) ccw projected
  arc A485 (-20.4754, 1.0044) -> (-20.4911, 0.6052) centre (0, 0) ccw projected
  arc A486 (-20.0133, 1.1629) -> (-20.4754, 1.0044) centre (-17.7834, -6.0894) ccw projected
  arc A487 (-19.633, 1.2671) -> (-20.0133, 1.1629) centre (-18.1301, -4.9618) ccw projected
  arc A488 (-19.3292, 1.331) -> (-19.633, 1.2671) centre (-18.3965, -3.8577) ccw projected
  arc A489 (-19.2995, 1.7091) -> (-19.3292, 1.331) centre (0, 0) ccw projected
  arc A490 (-19.5895, 1.8197) -> (-19.2995, 1.7091) centre (-17.5665, 6.6881) ccw projected
  arc A491 (-19.9489, 1.9822) -> (-19.5895, 1.8197) centre (-17.1307, 7.7369) ccw projected
  arc A492 (-20.3804, 2.2111) -> (-19.9489, 1.9822) centre (-16.6119, 8.7963) ccw projected
  arc A493 (-20.3335, 2.6078) -> (-20.3804, 2.2111) centre (0, 0) ccw projected
  arc A494 (-19.8604, 2.7295) -> (-20.3335, 2.6078) centre (-18.2064, -4.6753) ccw projected
  arc A495 (-19.473, 2.8036) -> (-19.8604, 2.7295) centre (-18.4635, -3.5241) ccw projected
  arc A496 (-19.1652, 2.8435) -> (-19.473, 2.8036) centre (-18.6425, -2.4025) ccw projected
  arc A497 (-19.1059, 3.2181) -> (-19.1652, 2.8435) centre (0, 0) ccw projected
  arc A498 (-19.3863, 3.3511) -> (-19.1059, 3.2181) centre (-16.9876, 8.0457) ccw projected
  arc A499 (-19.7318, 3.5413) -> (-19.3863, 3.3511) centre (-16.4708, 9.0571) ccw projected
  arc A500 (-20.1441, 3.8033) -> (-19.7318, 3.5413) centre (-15.8705, 10.0726) ccw projected
  arc A501 (-20.0662, 4.1951) -> (-20.1441, 3.8033) centre (0, 0) ccw projected
  arc A502 (-19.585, 4.2793) -> (-20.0662, 4.1951) centre (-18.517, -3.2324) ccw projected
  arc A503 (-19.193, 4.3228) -> (-19.585, 4.2793) centre (-18.6831, -2.0646) ccw projected
  arc A504 (-18.883, 4.3384) -> (-19.193, 4.3228) centre (-18.7735, -0.9324) ccw projected
  arc A505 (-18.7945, 4.7072) -> (-18.883, 4.3384) centre (0, 0) ccw projected
  arc A506 (-19.0636, 4.8618) -> (-18.7945, 4.7072) centre (-16.304, 9.3537) ccw projected
  arc A507 (-19.3932, 5.0785) -> (-19.0636, 4.8618) centre (-15.7095, 10.3215) ccw projected
  arc A508 (-19.7836, 5.372) -> (-19.3932, 5.0785) centre (-15.0313, 11.2867) ccw projected
  arc A509 (-19.6752, 5.7565) -> (-19.7836, 5.372) centre (0, 0) ccw projected
  arc A510 (-19.1889, 5.8028) -> (-19.6752, 5.7565) centre (-18.7136, -1.7696) ccw projected
  arc A511 (-18.7947, 5.8154) -> (-19.1889, 5.8028) centre (-18.7875, -0.5924) ccw projected
  arc A512 (-18.4844, 5.8066) -> (-18.7947, 5.8154) centre (-18.7888, 0.5434) ccw projected
  arc A513 (-18.3672, 6.1673) -> (-18.4844, 5.8066) centre (0, 0) ccw projected
  arc A514 (-18.6234, 6.3425) -> (-18.3672, 6.1673) centre (-15.5199, 10.6041) ccw projected
  arc A515 (-18.9349, 6.5844) -> (-18.6234, 6.3425) centre (-14.8512, 11.5222) ccw projected
  arc A516 (-19.3011, 6.9077) -> (-18.9349, 6.5844) centre (-14.0994, 12.4312) ccw projected
  arc A517 (-19.1629, 7.2825) -> (-19.3011, 6.9077) centre (0, 0) ccw projected
  arc A518 (-18.6745, 7.2904) -> (-19.1629, 7.2825) centre (-18.7947, -0.2959) ccw projected
  arc A519 (-18.2805, 7.272) -> (-18.6745, 7.2904) centre (-18.776, 0.8835) ccw projected
  arc A520 (-17.9719, 7.2389) -> (-18.2805, 7.272) centre (-18.6882, 2.0159) ccw projected
  arc A521 (-17.8267, 7.5893) -> (-17.9719, 7.2389) centre (0, 0) ccw projected
  arc A522 (-18.0684, 7.7842) -> (-17.8267, 7.5893) centre (-14.64, 11.7891) ccw projected
  arc A523 (-18.36, 8.0497) -> (-18.0684, 7.7842) centre (-13.9014, 12.6519) ccw projected
  arc A524 (-18.6997, 8.4007) -> (-18.36, 8.0497) centre (-13.0806, 13.4991) ccw projected
  arc A525 (-18.5324, 8.7635) -> (-18.6997, 8.4007) centre (0, 0) ccw projected
  arc A526 (-18.0449, 8.7331) -> (-18.5324, 8.7635) centre (-18.76, 1.1796) ccw projected
  arc A527 (-17.6536, 8.6839) -> (-18.0449, 8.7331) centre (-18.6488, 2.3539) ccw projected
  arc A528 (-17.3485, 8.6267) -> (-17.6536, 8.6839) centre (-18.4724, 3.476) ccw projected
  arc A529 (-17.1763, 8.9646) -> (-17.3485, 8.6267) centre (0, 0) ccw projected
  arc A530 (-17.4019, 9.1778) -> (-17.1763, 8.9646) centre (-13.6699, 12.9014) ccw projected
  arc A531 (-17.6718, 9.4654) -> (-17.4019, 9.1778) centre (-12.8659, 13.7036) ccw projected
  arc A532 (-17.9829, 9.842) -> (-17.6718, 9.4654) centre (-11.9812, 14.4838) ccw projected
  arc A533 (-17.7877, 10.1905) -> (-17.9829, 9.842) centre (0, 0) ccw projected
  arc A534 (-17.3041, 10.122) -> (-17.7877, 10.1905) centre (-18.6096, 2.6478) ccw projected
  arc A535 (-16.9178, 10.0422) -> (-17.3041, 10.122) centre (-18.4067, 3.8099) ccw projected
  arc A536 (-16.6182, 9.9612) -> (-16.9178, 10.0422) centre (-18.1428, 4.9146) ccw projected
  arc A537 (-16.42, 10.2846) -> (-16.6182, 9.9612) centre (0, 0) ccw projected
  arc A538 (-16.6282, 10.5148) -> (-16.42, 10.2846) centre (-12.6156, 13.9341) ccw projected
  arc A539 (-16.8747, 10.8227) -> (-16.6282, 10.5148) centre (-11.7511, 14.6708) ccw projected
  arc A540 (-17.1553, 11.2226) -> (-16.8747, 10.8227) centre (-10.8078, 15.3792) ccw projected
  arc A541 (-16.9334, 11.5547) -> (-17.1553, 11.2226) centre (0, 0) ccw projected
  arc A542 (-16.4566, 11.4485) -> (-16.9334, 11.5547) centre (-18.3445, 4.0998) ccw projected
  arc A543 (-16.0778, 11.3386) -> (-16.4566, 11.4485) centre (-18.051, 5.2423) ccw projected
  arc A544 (-15.7854, 11.2344) -> (-16.0778, 11.3386) centre (-17.7012, 6.3229) ccw projected
  arc A545 (-15.5625, 11.5412) -> (-15.7854, 11.2344) centre (0, 0) ccw projected
  arc A546 (-15.752, 11.7871) -> (-15.5625, 11.5412) centre (-11.4834, 14.881) ccw projected
  arc A547 (-15.9735, 12.1134) -> (-15.752, 11.7871) centre (-10.5638, 15.5476) ccw projected
  arc A548 (-16.2219, 12.534) -> (-15.9735, 12.1134) centre (-9.5679, 16.1798) ccw projected
  arc A549 (-15.9746, 12.8477) -> (-16.2219, 12.534) centre (0, 0) ccw projected
  arc A550 (-15.5076, 12.7043) -> (-15.9746, 12.8477) centre (-17.9663, 5.5264) ccw projected
  arc A551 (-15.1386, 12.5651) -> (-15.5076, 12.7043) centre (-17.5841, 6.6424) ccw projected
  arc A552 (-14.8553, 12.4383) -> (-15.1386, 12.5651) centre (-17.1506, 7.6922) ccw projected
  arc A553 (-14.609, 12.7266) -> (-14.8553, 12.4383) centre (0, 0) ccw projected
  arc A554 (-14.7786, 12.9866) -> (-14.609, 12.7266) centre (-10.2805, 15.7361) ccw projected
  arc A555 (-14.9739, 13.3293) -> (-14.7786, 12.9866) centre (-9.3114, 16.3285) ccw projected
  arc A556 (-15.1885, 13.7681) -> (-14.9739, 13.3293) centre (-8.2689, 16.8806) ccw projected
  arc A557 (-14.9173, 14.0614) -> (-15.1885, 13.7681) centre (0, 0) ccw projected
  arc A558 (-14.463, 13.8819) -> (-14.9173, 14.0614) centre (-17.4773, 6.919) ccw projected
  arc A559 (-14.1061, 13.7141) -> (-14.463, 13.8819) centre (-17.0087, 8.0015) ccw projected
  arc A560 (-13.8336, 13.5655) -> (-14.1061, 13.7141) centre (-16.4942, 9.0141) ccw projected
  arc A561 (-13.5655, 13.8336) -> (-13.8336, 13.5655) centre (0, 0) ccw projected
  arc A562 (-13.7141, 14.1061) -> (-13.5655, 13.8336) centre (-9.0141, 16.4942) ccw projected
  arc A563 (-13.8819, 14.463) -> (-13.7141, 14.1061) centre (-8.0015, 17.0087) ccw projected
  arc A564 (-14.0614, 14.9173) -> (-13.8819, 14.463) centre (-6.919, 17.4773) ccw projected
  arc A565 (-13.7681, 15.1885) -> (-14.0614, 14.9173) centre (0, 0) ccw projected
  arc A566 (-13.3293, 14.9739) -> (-13.7681, 15.1885) centre (-16.8806, 8.2689) ccw projected
  arc A567 (-12.9866, 14.7786) -> (-13.3293, 14.9739) centre (-16.3285, 9.3114) ccw projected
  arc A568 (-12.7266, 14.609) -> (-12.9866, 14.7786) centre (-15.7361, 10.2805) ccw projected
  arc A569 (-12.4383, 14.8553) -> (-12.7266, 14.609) centre (0, 0) ccw projected
  arc A570 (-12.5651, 15.1386) -> (-12.4383, 14.8553) centre (-7.6922, 17.1506) ccw projected
  arc A571 (-12.7043, 15.5076) -> (-12.5651, 15.1386) centre (-6.6424, 17.5841) ccw projected
  arc A572 (-12.8477, 15.9746) -> (-12.7043, 15.5076) centre (-5.5264, 17.9663) ccw projected
  arc A573 (-12.534, 16.2219) -> (-12.8477, 15.9746) centre (0, 0) ccw projected
  arc A574 (-12.1134, 15.9735) -> (-12.534, 16.2219) centre (-16.1798, 9.5679) ccw projected
  arc A575 (-11.7871, 15.752) -> (-12.1134, 15.9735) centre (-15.5476, 10.5638) ccw projected
  arc A576 (-11.5412, 15.5625) -> (-11.7871, 15.752) centre (-14.881, 11.4834) ccw projected
  arc A577 (-11.2344, 15.7854) -> (-11.5412, 15.5625) centre (0, 0) ccw projected
  arc A578 (-11.3386, 16.0778) -> (-11.2344, 15.7854) centre (-6.3229, 17.7012) ccw projected
  arc A579 (-11.4485, 16.4566) -> (-11.3386, 16.0778) centre (-5.2423, 18.051) ccw projected
  arc A580 (-11.5547, 16.9334) -> (-11.4485, 16.4566) centre (-4.0998, 18.3445) ccw projected
  arc A581 (-11.2226, 17.1553) -> (-11.5547, 16.9334) centre (0, 0) ccw projected
  arc A582 (-10.8227, 16.8747) -> (-11.2226, 17.1553) centre (-15.3792, 10.8078) ccw projected
  arc A583 (-10.5148, 16.6282) -> (-10.8227, 16.8747) centre (-14.6708, 11.7511) ccw projected
  arc A584 (-10.2846, 16.42) -> (-10.5148, 16.6282) centre (-13.9341, 12.6156) ccw projected
  arc A585 (-9.9612, 16.6182) -> (-10.2846, 16.42) centre (0, 0) ccw projected
  arc A586 (-10.0422, 16.9178) -> (-9.9612, 16.6182) centre (-4.9146, 18.1428) ccw projected
  arc A587 (-10.122, 17.3041) -> (-10.0422, 16.9178) centre (-3.8099, 18.4067) ccw projected
  arc A588 (-10.1905, 17.7877) -> (-10.122, 17.3041) centre (-2.6478, 18.6096) ccw projected
  arc A589 (-9.842, 17.9829) -> (-10.1905, 17.7877) centre (0, 0) ccw projected
  arc A590 (-9.4654, 17.6718) -> (-9.842, 17.9829) centre (-14.4838, 11.9812) ccw projected
  arc A591 (-9.1778, 17.4019) -> (-9.4654, 17.6718) centre (-13.7036, 12.8659) ccw projected
  arc A592 (-8.9646, 17.1763) -> (-9.1778, 17.4019) centre (-12.9014, 13.6699) ccw projected
  arc A593 (-8.6267, 17.3485) -> (-8.9646, 17.1763) centre (0, 0) ccw projected
  arc A594 (-8.6839, 17.6536) -> (-8.6267, 17.3485) centre (-3.476, 18.4724) ccw projected
  arc A595 (-8.7331, 18.0449) -> (-8.6839, 17.6536) centre (-2.3539, 18.6488) ccw projected
  arc A596 (-8.7635, 18.5324) -> (-8.7331, 18.0449) centre (-1.1796, 18.76) ccw projected
  arc A597 (-8.4007, 18.6997) -> (-8.7635, 18.5324) centre (0, 0) ccw projected
  arc A598 (-8.0497, 18.36) -> (-8.4007, 18.6997) centre (-13.4991, 13.0806) ccw projected
  arc A599 (-7.7842, 18.0684) -> (-8.0497, 18.36) centre (-12.6519, 13.9014) ccw projected
  arc A600 (-7.5893, 17.8267) -> (-7.7842, 18.0684) centre (-11.7891, 14.64) ccw projected
  arc A601 (-7.2389, 17.9719) -> (-7.5893, 17.8267) centre (0, 0) ccw projected
  arc A602 (-7.272, 18.2805) -> (-7.2389, 17.9719) centre (-2.0159, 18.6882) ccw projected
  arc A603 (-7.2904, 18.6745) -> (-7.272, 18.2805) centre (-0.8835, 18.776) ccw projected
  arc A604 (-7.2825, 19.1629) -> (-7.2904, 18.6745) centre (0.2959, 18.7947) ccw projected
  arc A605 (-6.9077, 19.3011) -> (-7.2825, 19.1629) centre (0, 0) ccw projected
  arc A606 (-6.5844, 18.9349) -> (-6.9077, 19.3011) centre (-12.4312, 14.0994) ccw projected
  arc A607 (-6.3425, 18.6234) -> (-6.5844, 18.9349) centre (-11.5222, 14.8512) ccw projected
  arc A608 (-6.1673, 18.3672) -> (-6.3425, 18.6234) centre (-10.6041, 15.5199) ccw projected
  arc A609 (-5.8066, 18.4844) -> (-6.1673, 18.3672) centre (0, 0) ccw projected
  arc A610 (-5.8154, 18.7947) -> (-5.8066, 18.4844) centre (-0.5434, 18.7888) ccw projected
  arc A611 (-5.8028, 19.1889) -> (-5.8154, 18.7947) centre (0.5924, 18.7875) ccw projected
  arc A612 (-5.7565, 19.6752) -> (-5.8028, 19.1889) centre (1.7696, 18.7136) ccw projected
  arc A613 (-5.372, 19.7836) -> (-5.7565, 19.6752) centre (0, 0) ccw projected
  arc A614 (-5.0785, 19.3932) -> (-5.372, 19.7836) centre (-11.2867, 15.0313) ccw projected
  arc A615 (-4.8618, 19.0636) -> (-5.0785, 19.3932) centre (-10.3215, 15.7095) ccw projected
  arc A616 (-4.7072, 18.7945) -> (-4.8618, 19.0636) centre (-9.3537, 16.304) ccw projected
  arc A617 (-4.3384, 18.883) -> (-4.7072, 18.7945) centre (0, 0) ccw projected
  arc A618 (-4.3228, 19.193) -> (-4.3384, 18.883) centre (0.9324, 18.7735) ccw projected
  arc A619 (-4.2793, 19.585) -> (-4.3228, 19.193) centre (2.0646, 18.6831) ccw projected
  arc A620 (-4.1951, 20.0662) -> (-4.2793, 19.585) centre (3.2324, 18.517) ccw projected
  arc A621 (-3.8033, 20.1441) -> (-4.1951, 20.0662) centre (0, 0) ccw projected
  arc A622 (-3.5413, 19.7318) -> (-3.8033, 20.1441) centre (-10.0726, 15.8705) ccw projected
  arc A623 (-3.3511, 19.3863) -> (-3.5413, 19.7318) centre (-9.0571, 16.4708) ccw projected
  arc A624 (-3.2181, 19.1059) -> (-3.3511, 19.3863) centre (-8.0457, 16.9876) ccw projected
  arc A625 (-2.8435, 19.1652) -> (-3.2181, 19.1059) centre (0, 0) ccw projected
  arc A626 (-2.8036, 19.473) -> (-2.8435, 19.1652) centre (2.4025, 18.6425) ccw projected
  arc A627 (-2.7295, 19.8604) -> (-2.8036, 19.473) centre (3.5241, 18.4635) ccw projected
  arc A628 (-2.6078, 20.3335) -> (-2.7295, 19.8604) centre (4.6753, 18.2064) ccw projected
  arc A629 (-2.2111, 20.3804) -> (-2.6078, 20.3335) centre (0, 0) ccw projected
  arc A630 (-1.9822, 19.9489) -> (-2.2111, 20.3804) centre (-8.7963, 16.6119) ccw projected